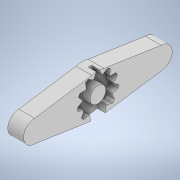
# Autodesk Inventor part: servo horn
Saved by Autodesk Inventor 2021 (Build 250183000, 183)
## iProperties
Created: 2025-04-02
Part Number: servo horn
Material: Generic
Document SubType Name: Modeling
Designer: Admin
Density: 1 g/cm^3
Appearance: Default
Author: Admin
Autodesk Inventor part; units mm, degrees
ref_plane "YZ Plane" through (0, 0, 0) normal (1, 0, 0) x (0, 1, 0)
ref_plane "XZ Plane" through (0, 0, 0) normal (0, 1, 0) x (-1, 0, 0)
ref_plane "XY Plane" through (0, 0, 0) normal (0, 0, 1) x (1, 0, 0)
sketch "Sketch1" plane through (0, 0, 0) normal (1, 0, 0) x (0, 1, 0)
  arc A0 (3.5, 20) -> (-3.5, 20) centre (0, 20) ccw
  line L0 (6.2139, 1.9071) -> (3.5, 20)
  line L1 (-3.5, 20) -> (-6.2139, 1.9071)
  line L2 (0, 0) -> (2.6706, 0)
  arc A1 (-3.5, -20) -> (3.5, -20) centre (0, -20) ccw
  line L3 (-3.5, -20) -> (-6.2139, -1.9071)
  line L4 (6.2139, -1.9071) -> (3.5, -20)
  arc A2 (-6.2139, 1.9071) -> (-6.2139, -1.9071) centre (0, 0) ccw
  arc A3 (6.2139, -1.9071) -> (6.2139, 1.9071) centre (0, 0) ccw
  line L5 (0, 0) -> (2.6706, 0)
  point P0 (6.5, 0)
  point P1 (-6.5, 0)
  dimension "d0" = 7
  dimension "d1" = 20
  constraints: 12 end point, 10 point on circle, 4 centre point, 3 symmetric about line, 2 horizontal, 1 other
  measures "d0" diameter of A0
  measures "d1" distance of A0.centre L2.start
extrude "Extrusion1" add sketch "Sketch1" along normal blind 5
sketch "Sketch2" plane through (5, 0, 0) normal (1, 0, 0) x (0, 0, -1)
  line L0 (0, 6.5) -> (0.5, 6.5)
  line L1 (0.5, 6.5) -> (1.2768, 4.8342)
  line L2 (-0.5, 6.5) -> (-1.2768, 4.8342)
  line L3 (0, 6.5) -> (-0.5, 6.5)
  line L4 (-3.5142, 5.4681) -> (-3.0935, 5.7385)
  line L5 (-3.0935, 5.7385) -> (-1.5395, 4.7571)
  line L6 (-3.9348, 5.1978) -> (-3.6877, 3.3766)
  line L7 (-3.5142, 5.4681) -> (-3.9348, 5.1978)
  line L8 (-5.9126, 2.7002) -> (-5.7049, 3.155)
  line L9 (-5.7049, 3.155) -> (-3.867, 3.1696)
  line L10 (-6.1203, 2.2454) -> (-4.9278, 0.8468)
  line L11 (-5.9126, 2.7002) -> (-6.1203, 2.2454)
  line L12 (-6.4338, -0.925) -> (-6.505, -0.4301)
  line L13 (-6.505, -0.4301) -> (-4.9667, 0.5758)
  line L14 (-6.3627, -1.42) -> (-4.6033, -1.9517)
  line L15 (-6.4338, -0.925) -> (-6.3627, -1.42)
  line L16 (-4.9124, -4.2566) -> (-5.2398, -3.8787)
  line L17 (-5.2398, -3.8787) -> (-4.4896, -2.2008)
  line L18 (-4.5849, -4.6345) -> (-2.8174, -4.1307)
  line L19 (-4.9124, -4.2566) -> (-4.5849, -4.6345)
  line L20 (-1.8313, -6.2367) -> (-2.311, -6.0958)
  line L21 (-2.311, -6.0958) -> (-2.587, -4.2787)
  line L22 (-1.3515, -6.3776) -> (-0.1369, -4.9981)
  line L23 (-1.8313, -6.2367) -> (-1.3515, -6.3776)
  line L24 (1.8313, -6.2367) -> (1.3515, -6.3776)
  line L25 (1.3515, -6.3776) -> (0.1369, -4.9981)
  line L26 (2.311, -6.0958) -> (2.587, -4.2787)
  line L27 (1.8313, -6.2367) -> (2.311, -6.0958)
  line L28 (4.9124, -4.2566) -> (4.5849, -4.6345)
  line L29 (4.5849, -4.6345) -> (2.8174, -4.1307)
  line L30 (5.2398, -3.8787) -> (4.4896, -2.2008)
  line L31 (4.9124, -4.2566) -> (5.2398, -3.8787)
  line L32 (6.4338, -0.925) -> (6.3627, -1.42)
  line L33 (6.3627, -1.42) -> (4.6033, -1.9517)
  line L34 (6.505, -0.4301) -> (4.9667, 0.5758)
  line L35 (6.4338, -0.925) -> (6.505, -0.4301)
  line L36 (5.9126, 2.7002) -> (6.1203, 2.2454)
  line L37 (6.1203, 2.2454) -> (4.9278, 0.8468)
  line L38 (5.7049, 3.155) -> (3.867, 3.1696)
  line L39 (5.9126, 2.7002) -> (5.7049, 3.155)
  line L40 (3.5142, 5.4681) -> (3.9348, 5.1978)
  line L41 (3.9348, 5.1978) -> (3.6877, 3.3766)
  line L42 (3.0935, 5.7385) -> (1.5395, 4.7571)
  line L43 (3.5142, 5.4681) -> (3.0935, 5.7385)
  arc A0 (-1.2768, 4.8342) -> (-1.5395, 4.7571) centre (0, 0) ccw
  arc A1 (1.5395, 4.7571) -> (1.2768, 4.8342) centre (0, 0) ccw
  arc A2 (3.867, 3.1696) -> (3.6877, 3.3766) centre (0, 0) ccw
  arc A3 (4.9667, 0.5758) -> (4.9278, 0.8468) centre (0, 0) ccw
  arc A4 (4.4896, -2.2008) -> (4.6033, -1.9517) centre (0, 0) ccw
  arc A5 (2.587, -4.2787) -> (2.8174, -4.1307) centre (0, 0) ccw
  arc A6 (-0.1369, -4.9981) -> (0.1369, -4.9981) centre (0, 0) ccw
  arc A7 (-2.8174, -4.1307) -> (-2.587, -4.2787) centre (0, 0) ccw
  arc A8 (-4.6033, -1.9517) -> (-4.4896, -2.2008) centre (0, 0) ccw
  arc A9 (-3.6877, 3.3766) -> (-3.867, 3.1696) centre (0, 0) ccw
  arc A10 (-4.9278, 0.8468) -> (-4.9667, 0.5758) centre (0, 0) ccw
  circle A11 centre (0, 0) radius 2.5
  arc A12 (-1.9071, -6.2139) -> (1.9071, -6.2139) centre (0, 0) ccw projected
  line L44 (-2.311, -6.0958) -> (-2.3021, -6.1547)
  line L45 (-20, -3.5) -> (-1.9071, -6.2139) projected
  line L46 (-2.3021, -6.1547) -> (-1.9071, -6.2139)
  line L47 (2.311, -6.0958) -> (2.3021, -6.1547)
  line L48 (1.9071, -6.2139) -> (20, -3.5) projected
  line L49 (2.3021, -6.1547) -> (1.9088, -6.2139)
  arc A13 (-6.4865, -0.4181) -> (-6.4338, -0.925) centre (0, 0) ccw
  arc A14 (-5.2308, -3.8586) -> (-4.9124, -4.2566) centre (0, 0) ccw
  arc A15 (-2.3143, -6.074) -> (-1.3369, -6.361) centre (0, 0) ccw
  arc A16 (0, -6.5) -> (2.3143, -6.074) centre (0, 0) ccw
  point P0 (0, 5)
  point P1 (-2.7032, 4.2063)
  point P2 (-4.5482, 2.0771)
  point P3 (-4.9491, -0.7116)
  point P4 (-3.7787, -3.2743)
  point P5 (-1.4087, -4.7975)
  point P6 (1.4087, -4.7975)
  point P7 (3.7787, -3.2743)
  point P8 (4.9491, -0.7116)
  point P9 (4.5482, 2.0771)
  point P10 (2.7032, 4.2063)
  dimension "d8" = 0.5
  dimension "d9" = 115
  dimension "d10" = 6.5
  dimension "d11" = 360
  dimension "d12" = 5
  constraints: 96 end point, 32 point on circle, 16 centre point, 8 point on line, 1 coincident, 1 horizontal, 111 other
  measures "d8" distance of L0.start L0.end
  measures "d9" angle of L0 L1
  measures "d10" distance from line of A0.centre L3
  measures "d12" diameter of A11
extrude "Extrusion2" cut sketch "Sketch2" against normal blind 2.5 contours L0 L1 A1 L42 L43 L40 L41 A2 L38 L39 L36 L37 A3 L34 L35 L32 L33 A4 L30 L31 L28 L29 A5 L26 A16 L27 A12 L25 A6 L22 L20 A15 L21 A7 L18 L19 A14 L17 A8 L14 L15 A13 L13 A10 L10 L11 L8 L9 A9 L6 L7 L4 L5 A0 L2 L3 | L26 L27 A16 | A15 L20 L21 | L47 L48 L27 | L20 L45 L44 | A12 L22 A6 L25
body "Solid1"
